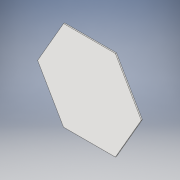
# Autodesk Inventor part: Frosted Top v1
Saved by Autodesk Inventor 2019 (Build 230136000, 136)
## iProperties
Created: 2021-07-14
Part Number: Frosted Top v1
Material: Generic
Document SubType Name: Modeling
Designer: Lix
Density: 1 g/cm^3
Appearance: White
Author: Lix
Autodesk Inventor part; units mm, degrees
ref_plane "YZ Plane" through (0, 0, 0) normal (1, 0, 0) x (0, 1, 0)
ref_plane "XZ Plane" through (0, 0, 0) normal (0, 1, 0) x (-1, 0, 0)
ref_plane "XY Plane" through (0, 0, 0) normal (0, 0, 1) x (1, 0, 0)
sketch "Sketch1" plane through (0, 0, 0) normal (0, 0, 1) x (1, 0, 0)
  line L0 (-47.9201, 83) -> (47.9201, 83)
  line L1 (47.9201, 83) -> (95.8401, 0)
  line L2 (95.8401, 0) -> (47.9201, -83)
  line L3 (47.9201, -83) -> (-47.9201, -83)
  line L4 (-47.9201, -83) -> (-95.8401, 0)
  line L5 (-95.8401, 0) -> (-47.9201, 83)
  point P0 (0, 0)
  point P1 (0, 0)
  dimension "d0" = 166
  constraints: 12 end point, 1 coincident, 1 horizontal, 13 other
  measures "d0" distance between parallel lines of L4 L1
extrude "Extrusion1" add sketch "Sketch1" along normal blind 2
sketch "Sketch3" plane through (0, 0, 2) normal (0, 0, 1) x (1, 0, 0)
  line L0 (47.9201, 83) -> (-47.9201, 83) projected
  line L1 (-47.9201, 83) -> (-95.8401, 0) projected
  line L2 (-95.8401, 0) -> (-47.9201, -83) projected
  line L3 (-47.9201, -83) -> (47.9201, -83) projected
  line L4 (47.9201, -83) -> (95.8401, 0) projected
  line L5 (95.8401, 0) -> (47.9201, 83) projected
  line L6 (-95.8401, 83) -> (95.8401, 83)
  line L7 (95.8401, 83) -> (95.8401, -83)
  line L8 (95.8401, -83) -> (-95.8401, -83)
  line L9 (-95.8401, -83) -> (-95.8401, 83)
  line L10 (-95.8401, 83) -> (95.8401, -83) construction
  line L11 (95.8401, 83) -> (-95.8401, -83) construction
  point P0 (0, 0)
  dimension "d3" = 191.6803
  dimension "d4" = 166
  constraints: 12 end point, 3 midpoint, 2 parallel, 1 collinear, 1 horizontal, 1 perpendicular
  measures "d3" distance of L6.start L6.end
  measures "d4" distance of L6.end L7.end
body "Solid1"
